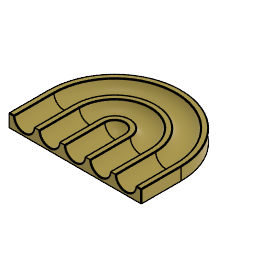
Sponge Holder (Autodesk Fusion 360 design; units mm, degrees)
Autodesk Fusion 360 part; units mm, degrees
sketch "Reference photo guestimated dimensions" plane through (0, 0, 0) normal (0, 1, 0) x (1, 0, 0)
  line L0 (-50.1946, -42.0047) -> (36.7426, 8.5183)
  line L1 (-49.4291, -51.7654) -> (38.9378, -0.4115)
  line L2 (38.9378, -0.4115) -> (36.7426, 8.5183)
  line L3 (-50.1946, -42.0047) -> (-49.4291, -51.7654)
  line L4 (-45.94, -50.8799) -> (-33.1803, -43.4648)
  line L5 (-33.1803, -43.4648) -> (-30.1867, -41.725)
  line L6 (-30.1867, -41.725) -> (-16.8124, -33.9526)
  line L7 (-16.8124, -33.9526) -> (-13.9011, -32.2608)
  line L8 (-13.9011, -32.2608) -> (0.2473, -24.0385)
  line L9 (0.2473, -24.0385) -> (3.4341, -22.1865)
  dimension "d6" = 100.5517
  dimension "d7" = 9.7607
  dimension "d8" = 14.7578
  dimension "d9" = 3.4624
  dimension "d10" = 15.4688
  dimension "d11" = 3.3671
  dimension "d12" = 16.3641
  constraint parallel L0 L1
  constraint parallel L1 L4
  constraint parallel L4 L5
  constraint parallel L1 L6
  constraint parallel L6 L7
  constraint parallel L1 L8
  constraint parallel L8 L9
  measures "d6" distance of L0.start L0.end
  measures "d7" vertical distance of L0.start L1.start
  measures "d8" distance of L4.start L4.end
  measures "d9" distance of L4.end L5.end
  measures "d10" distance of L5.end L6.end
  measures "d11" distance of L6.end L7.end
  measures "d12" distance of L7.end L8.end
sketch "Body Sketch" plane through (0, 0, 0) normal (0, 0, 1) x (1, 0, 0)
  arc A0 (50, 0) -> (-50, 0) centre (0, 0) ccw
  line L0 (0, 0) -> (0, 16.4772)
  line L1 (-50, 0) -> (-50, -30)
  line L2 (50, 0) -> (50, -30)
  line L3 (-50, -30) -> (50, -30)
  point P0 (0, 50)
  dimension "d1" = 100
  dimension "d3" = 80
  constraint coincident A0.centre L0.start
  constraint vertical L0
  constraint tangent A0 L1
  constraint vertical L1
  constraint symmetric A0.end L0 A0.start
  constraint symmetric L0 L1.end L2.end
  constraint midpoint A0 P0
  measures "d1" distance of L1.end L2.end
  measures "d3" vertical distance of L1.end P0
extrude "Extrude1" add sketch "Body Sketch" against normal blind 10
sketch "Paths" plane through (0, 0, 0) normal (0, 0, 1) x (-1, 0, 0)
  arc A0 (-50, 0) -> (50, 0) centre (0, 0) ccw
  line L0 (50, 0) -> (50, 30)
  line L1 (50, 30) -> (-50, 30)
  line L2 (-50, 30) -> (-50, 0)
  line L3 (0, 30) -> (0, 0)
  line L4 (19.1667, 30) -> (19.1667, 0)
  line L5 (38.3333, 30) -> (38.3333, 0)
  line L6 (-38.3333, 30) -> (-38.3333, 0)
  line L7 (-19.1667, 30) -> (-19.1667, 0)
  arc A1 (-38.3333, 0) -> (38.3333, 0) centre (0, 0) ccw
  arc A2 (-19.1667, 0) -> (19.1667, 0) centre (0, 0) ccw
  circle A3 centre (0, 30) radius 7.5 construction
  line L8 (30.8333, 65.11) -> (26.6667, 65.11)
  line L9 (26.6667, 65.11) -> (11.6667, 65.11) construction
  line L10 (11.6667, 65.11) -> (7.5, 65.11)
  line L11 (50, 65.11) -> (45.8333, 65.11)
  line L12 (45.8333, 65.11) -> (30.8333, 65.11) construction
  line L13 (7.5, 65.11) -> (0, 65.11) construction
  line L14 (38.3333, 65.11) -> (38.3333, 61.0465) construction
  line L15 (19.1667, 65.11) -> (19.1667, 61.3275) construction
  line L16 (50, 30) -> (50, 65.11) construction
  dimension "d14" = 100
  dimension "d30" = 15
  dimension "d31" = 15
  dimension "d32" = 15
  dimension "d33" = 7.5
  dimension "d34" = 50
  dimension "d35" = 4.1667
  dimension "d36" = 11.6667
  dimension "d37" = 19.1667
  dimension "d38" = 7.5
  dimension "d39" = 7.5
  dimension "d40" = 4.1667
  dimension "d41" = 7.5
  constraint midpoint L1 L3.start
  constraint perpendicular L1 L3
  constraint coincident A0.centre L3.end
  constraint coincident L1 L4.start
  constraint perpendicular L1 L4
  constraint coincident L1 L5.start
  constraint perpendicular L1 L5
  constraint horizontal L4.end L5.end
  constraint horizontal A0.centre L4.end
  constraint symmetric L3 L4.start L7.start
  constraint symmetric L3 L4.end L7.end
  constraint symmetric L3 L5.start L6.start
  constraint symmetric L3 L5.end L6.end
  constraint coincident L3.start A3.centre
  constraint horizontal L8
  constraint parallel L8 L9
  constraint parallel L9 L10
  constraint equal L8 L10
  constraint horizontal L11
  constraint parallel L11 L12
  constraint coincident L8.start L12.end
  constraint horizontal L13
  constraint equal L8 L11
  constraint vertical L0.end L11.start
  constraint midpoint L12 L14.start
  constraint perpendicular L12 L14
  constraint midpoint L9 L15.start
  constraint perpendicular L9 L15
  constraint coincident L0.end L1.start
  measures "d14" distance of L0.end L1.end
  measures "d30" diameter of A3
  measures "d31" distance of L8.end L9.end
  measures "d32" distance of L11.end L8.start
  measures "d33" distance of L10.end L13.end
  measures "d34" distance of L11.start L13.end
  measures "d35" distance of L11.end L11.start
  measures "d36" distance of L0.end L5.start
  measures "d37" distance of L4.start L5.start
  measures "d38" distance of L11.end L14.start
  measures "d39" distance of L8.start L14.start
  measures "d40" distance of L8.start L8.end
  measures "d41" distance of L8.end L15.start
pipe "Pipe1" cut diameter 15 path "Paths" along L5 A1 L6
pipe "Pipe2" cut diameter 15 path "Paths" along L4 A2 L7
pipe "Pipe3" cut diameter 15 path "Paths" along L3
revolve "Revolve1" cut 1 faces at (-0.5563, 0, -2.4373) angle 360 about axis through (-7.5, 0, 0) along (1, 0, 0)
fillet "Fillet1" radius 0.4 2 edges at (-50, -30, -5) (50, -30, -5)
chamfer "Chamfer1" distance 0.4 angle 45 27 edges at (-50, -14.8, 0) (-49.8828, -29.8828, 0) (-47.7167, -30, 0) (47.7167, -30, 0) (49.8828, -29.8828, 0) (50, -14.8, 0) (0, 50, 0) (-45.8333, -15, 0) (0, 45.8333, 0) (45.8333, -15, 0) (-30.8333, -15, 0) (30.8333, -15, 0) (0, 30.8333, 0) (-26.6667, -15, 0) (0, 26.6667, 0) (26.6667, -15, 0) (-11.6667, -15, 0) (11.6667, -15, 0) (0, 11.6667, 0) (-7.5, -15, 0) (0, 7.5, 0) (7.5, -15, 0) (-38.3333, -30, -7.5) (-19.1667, -30, -7.5) (0, -30, -7.5) (19.1667, -30, -7.5) (38.3333, -30, -7.5) 1 faces at (-9.7977, 24.1492, -10)
equation "d15 = d14 / 6"
equation "d36 = d35 + 7.5 mm"
equation "d37 = d35 + 15 mm"
